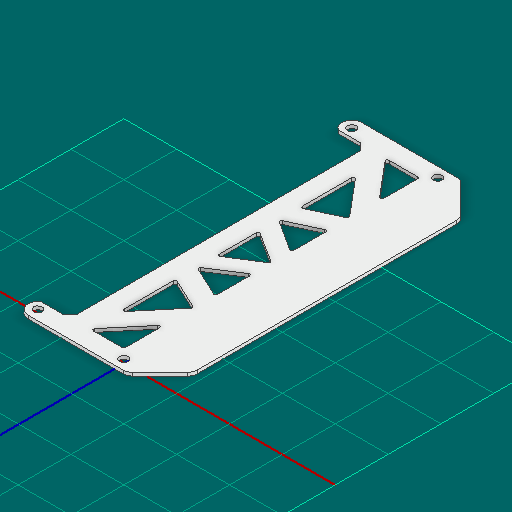
# Autodesk Inventor part: ramp
Saved by Autodesk Inventor 2025 (Build 290162000, 162)
## iProperties
Created: 2024-08-22
Part Number: ramp
Material: Acetal Resin, White
Document SubType Name: Modeling
Designer: averey
Density: 1.425 g/cm^3
Appearance: Smooth - White
Author: averey
Autodesk Inventor part; units mm, degrees
ref_plane "YZ Plane" through (0, 0, 0) normal (1, 0, 0) x (0, 1, 0)
ref_plane "XZ Plane" through (0, 0, 0) normal (0, 1, 0) x (-1, 0, 0)
ref_plane "XY Plane" through (0, 0, 0) normal (0, 0, 1) x (1, 0, 0)
sketch "Sketch1" plane through (0, 0, 0) normal (0, 1, 0) x (-1, 0, 0)
  circle A0 centre (0, 0) radius 2.0955
  circle A1 centre (41.2753, 0) radius 2.0955
  circle A2 centre (0, -150.8125) radius 2.0955
  circle A3 centre (41.2753, -150.8125) radius 2.0955
  arc A4 (43.9079, -3.9688) -> (41.2753, 4.7625) centre (41.2753, 0) ccw
  arc A5 (41.2753, -155.575) -> (43.9079, -146.8438) centre (41.2753, -150.8125) ccw
  line L0 (29.8453, -7.366) -> (29.8453, -143.4465)
  line L1 (41.2753, -155.575) -> (0, -155.575)
  line L2 (0, 4.7625) -> (41.2753, 4.7625)
  line L3 (33.2426, -3.9688) -> (29.8453, -7.366)
  line L4 (29.8453, -143.4465) -> (33.2426, -146.8438)
  line L5 (18.9991, -146.431) -> (5.1753, -146.431)
  line L6 (5.1753, -4.3815) -> (18.9991, -4.3815)
  line L7 (19.6072, -5.6855) -> (5.7833, -22.1601)
  line L8 (20.7013, -4.3815) -> (42.2074, -4.3815) construction
  line L9 (19.2995, -20.2776) -> (5.0464, -37.2638)
  line L10 (5.319, -38.4934) -> (19.5721, -45.1397)
  line L11 (4.3815, -38.0562) -> (20.108, -38.0562) construction
  line L12 (19.3974, -55.1476) -> (5.5107, -48.6721)
  line L13 (5.6049, -65.4746) -> (19.4917, -56.5343)
  line L14 (19.6072, -145.127) -> (5.7833, -128.6524)
  line L15 (20.7013, -146.431) -> (42.2074, -146.431) construction
  line L16 (19.2995, -130.5349) -> (5.0464, -113.5487)
  line L17 (5.319, -112.3191) -> (19.5721, -105.6728)
  line L18 (4.3815, -112.7563) -> (20.108, -112.7563) construction
  line L19 (19.3974, -95.6649) -> (5.5107, -102.1404)
  line L20 (19.4917, -94.2782) -> (5.6049, -85.3379)
  line L21 (20.7013, -95.0569) -> (37.217, -95.0569) construction
  line L22 (5.4426, -76.0771) -> (19.4834, -84.9549)
  line L23 (5.4426, -74.7354) -> (19.4834, -65.8576)
  line L24 (4.3815, -21.6499) -> (4.3815, -5.1753)
  line L25 (20.7013, -20.7878) -> (20.7013, -44.4203)
  line L26 (4.3815, -64.8072) -> (4.3815, -49.3915)
  line L27 (20.7013, -66.5285) -> (20.7013, -84.284)
  line L28 (20.7013, -106.3922) -> (20.7013, -130.0247)
  line L29 (4.3815, -145.6373) -> (4.3815, -129.1626)
  line L30 (4.3815, -101.421) -> (4.3815, -86.0053)
  arc A6 (4.3815, -21.6499) -> (5.7833, -22.1601) centre (5.1753, -21.6499) ccw
  arc A7 (5.1753, -4.3815) -> (4.3815, -5.1753) centre (5.1753, -5.1753) ccw
  arc A8 (19.6072, -5.6855) -> (18.9991, -4.3815) centre (18.9991, -5.1753) ccw
  arc A9 (20.7013, -20.7878) -> (19.2995, -20.2776) centre (19.9076, -20.7878) ccw
  arc A10 (5.0464, -37.2638) -> (5.319, -38.4934) centre (5.6545, -37.774) ccw
  arc A11 (19.5721, -45.1397) -> (20.7013, -44.4203) centre (19.9076, -44.4203) ccw
  arc A12 (5.5107, -48.6721) -> (4.3815, -49.3915) centre (5.1753, -49.3915) ccw
  arc A13 (4.3815, -64.8072) -> (5.6049, -65.4746) centre (5.1753, -64.8072) ccw
  arc A14 (19.4917, -56.5343) -> (19.3974, -55.1476) centre (19.062, -55.8669) ccw
  arc A15 (5.4426, -74.7354) -> (5.4426, -76.0771) centre (5.8668, -75.4063) ccw
  arc A16 (19.4834, -84.9549) -> (20.7013, -84.284) centre (19.9076, -84.284) ccw
  arc A17 (20.7013, -66.5285) -> (19.4834, -65.8576) centre (19.9076, -66.5285) ccw
  arc A18 (5.6049, -85.3379) -> (4.3815, -86.0053) centre (5.1753, -86.0053) ccw
  arc A19 (19.3974, -95.6649) -> (19.4917, -94.2782) centre (19.062, -94.9456) ccw
  arc A20 (4.3815, -101.421) -> (5.5107, -102.1404) centre (5.1753, -101.421) ccw
  arc A21 (20.7013, -106.3922) -> (19.5721, -105.6728) centre (19.9076, -106.3922) ccw
  arc A22 (5.319, -112.3191) -> (5.0464, -113.5487) centre (5.6545, -113.0385) ccw
  arc A23 (19.2995, -130.5349) -> (20.7013, -130.0247) centre (19.9076, -130.0247) ccw
  arc A24 (5.7833, -128.6524) -> (4.3815, -129.1626) centre (5.1753, -129.1626) ccw
  arc A25 (4.3815, -145.6373) -> (5.1753, -146.431) centre (5.1753, -145.6373) ccw
  arc A26 (18.9991, -146.431) -> (19.6072, -145.127) centre (18.9991, -145.6373) ccw
  line L31 (0, 4.7625) -> (-4.3773, 4.7625)
  line L32 (-22.225, -13.0852) -> (-22.225, -137.7273)
  line L33 (-4.3773, -155.575) -> (0, -155.575)
  line L34 (43.9079, -3.9688) -> (33.2426, -3.9688)
  line L35 (43.9079, -146.8438) -> (33.2426, -146.8438)
  line L36 (-20.8301, -9.7176) -> (-7.7449, 3.3676)
  line L37 (-20.8301, -141.0949) -> (-7.7449, -154.1801)
  arc A27 (-4.3773, 4.7625) -> (-7.7449, 3.3676) centre (-4.3773, 0) ccw
  arc A28 (-20.8301, -9.7176) -> (-22.225, -13.0852) centre (-17.4625, -13.0852) ccw
  arc A29 (-22.225, -137.7273) -> (-20.8301, -141.0949) centre (-17.4625, -137.7273) ccw
  arc A30 (-7.7449, -154.1801) -> (-4.3773, -155.575) centre (-4.3773, -150.8125) ccw
  point P0 (29.8453, -4.7625)
  point P1 (29.8453, -146.05)
  point P2 (32.8298, -4.3815)
  point P3 (32.4488, -146.05)
  point P4 (-17.4625, 4.7625)
  point P5 (-22.225, 0)
  point P6 (-17.4625, -155.575)
  point P7 (-22.225, -150.8125)
  point P8 (-22.225, 4.7625)
  point P9 (-22.225, -11.1125)
  point P10 (-6.35, 4.7625)
  point P11 (-22.225, 4.7625)
  point P12 (-22.225, -139.7)
  point P13 (-6.35, -155.575)
  point P14 (-22.225, -155.575)
  dimension "d0" = 4.191
  dimension "d3" = 9.525
  dimension "d10" = 130
  dimension "d11" = 9.144
  dimension "d12" = 25
  dimension "d13" = 9.144
  dimension "d15" = 130
  dimension "d16" = 9.144
  dimension "d17" = 25
  dimension "d18" = 9.144
  dimension "d19" = 147.227
  dimension "d20" = 0.7937
  dimension "d24" = 22.225
  dimension "d27" = 15.875
  dimension "d28" = 15.875
  dimension "d29" = 15.875
  dimension "d30" = 15.875
  dimension "d31" = 4.7625
  constraints: 74 end point, 54 point on circle, 50 tangent, 31 centre point, 26 point on line, 23 equal radius, 8 horizontal, 5 equal length, 4 parallel, 3 coincident, 14 other
  measures "d0" diameter of A0
  measures "d3" diameter of A4
  measures "d10" angle of L7 L8
  measures "d11" distance between parallel lines of L7 L9
  measures "d12" angle of L10 L11
  measures "d13" distance between parallel lines of L10 L12
  measures "d15" angle of L15 L14
  measures "d16" distance between parallel lines of L14 L16
  measures "d17" angle of L18 L17
  measures "d18" distance between parallel lines of L17 L19
  measures "d19" angle of L21 L20
  measures "d20" radius of A6
  measures "d27" distance of point (-22.225, -11.113) point (-22.225, 4.762)
  measures "d28" distance of point (-6.35, 4.762) point (-22.225, 4.762)
  measures "d29" distance of point (-22.225, -139.7) point (-22.225, -155.575)
  measures "d30" distance of point (-6.35, -155.575) point (-22.225, -155.575)
  measures "d31" radius of A27
extrude "Extrusion1" add sketch "Sketch1" along normal blind 1.5875
equation "\"d28\" = d27"
equation "\"d29\" = d27"
equation "\"d30\" = d29"
body "Solid1"
